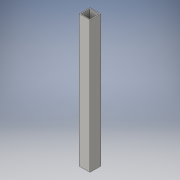
# Autodesk Inventor part: Main upright
Saved by Autodesk Inventor 2016 (Build 200138000, 138)
## iProperties
Created: 2017-11-09
Part Number: Main upright
Material: Generic
Document SubType Name: Modeling
Designer: thompson.nathaniel
Density: 1 g/cm^3
Appearance: Default
Author: thompson.nathaniel
Autodesk Inventor part; units mm, degrees
ref_plane "YZ Plane" through (0, 0, 0) normal (1, 0, 0) x (0, 1, 0)
ref_plane "XZ Plane" through (0, 0, 0) normal (0, 1, 0) x (-1, 0, 0)
ref_plane "XY Plane" through (0, 0, 0) normal (0, 0, 1) x (1, 0, 0)
sketch "Sketch1" plane through (0, 0, 0) normal (0, 1, 0) x (-1, 0, 0)
  line L0 (0, 0) -> (19.2484, 0)
  line L1 (19.2484, 0) -> (19.2484, -19.2484)
  line L2 (19.2484, -19.2484) -> (0, -19.2484)
  line L3 (0, -19.2484) -> (0, 0)
  line L4 (1.5875, -1.5875) -> (17.6609, -1.5875)
  line L5 (17.6609, -1.5875) -> (17.6609, -17.6609)
  line L6 (17.6609, -17.6609) -> (1.5875, -17.6609)
  line L7 (1.5875, -17.6609) -> (1.5875, -1.5875)
  dimension "d0" = 16.0734
  dimension "d1" = 1.5875
  dimension "d2" = 1.5875
  dimension "d3" = 1.5875
  dimension "d4" = 1.5875
  dimension "d5" = 16.0734
  constraints: 16 end point, 4 parallel, 2 horizontal, 2 perpendicular
  measures "d0" distance of L6.end L4.start
  measures "d1" distance between parallel lines of L4 L0
  measures "d2" distance between parallel lines of L2 L6
  measures "d3" distance between parallel lines of L5 L1
  measures "d4" distance between parallel lines of L3 L7
  measures "d5" distance between parallel lines of L7 L5
extrude "Extrusion1" add sketch "Sketch1" along normal blind 234.95
body "Solid1"
